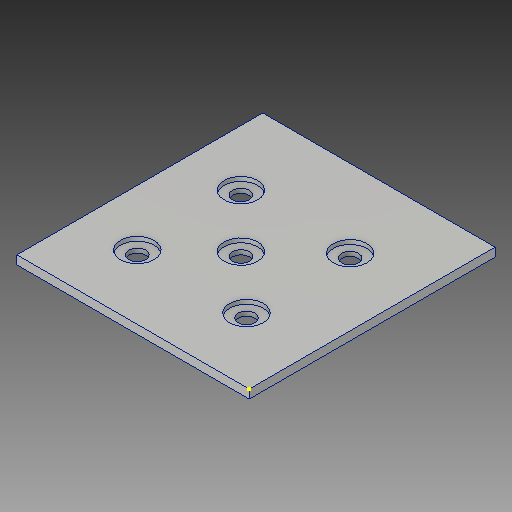
# Autodesk Inventor part: 底板
Saved by Autodesk Inventor 2017 (Build 210142000, 142)
## iProperties
Part Number: 底板
Material: 鋁合金 6061
Document SubType Name: Modeling
Designer: user
Density: 2.7 g/cm^3
Appearance: 鋁 - 平面
Author: user
Autodesk Inventor part; units mm, degrees
ref_plane "YZ Plane" through (0, 0, 0) normal (1, 0, 0) x (0, 1, 0)
ref_plane "XZ Plane" through (0, 0, 0) normal (0, 1, 0) x (-1, 0, 0)
ref_plane "XY Plane" through (0, 0, 0) normal (0, 0, 1) x (1, 0, 0)
sketch "草圖1" plane through (0, 0, 0) normal (0, 1, 0) x (-1, 0, 0)
  line L0 (0, 0) -> (83, 0)
  line L1 (83, 0) -> (83, -87.8)
  line L2 (83, -87.8) -> (0, -87.8)
  line L3 (0, -87.8) -> (0, 0)
  dimension "d0" = 87.8
  dimension "d1" = 83
  constraints: 8 end point, 2 parallel, 1 horizontal, 1 perpendicular
  measures "d0" distance of L0.end L1.end
  measures "d1" distance of L1.end L2.end
extrude "擠出1" add sketch "草圖1" along normal blind 3.1
sketch "草圖2" plane through (0, 3.1, 0) normal (0, 1, 0) x (1, 0, 0)
  line L0 (-24, -18.3432) -> (-24, 108.3328)
  line L1 (-63, -18.3432) -> (-63, 117.1807)
  line L2 (-93.8741, 60) -> (24.8173, 60)
  line L3 (19.8538, 23) -> (-101.6429, 23)
  line L4 (-44, -5.6109) -> (-44, 94.0899)
  line L5 (-89.7738, 41) -> (11.6533, 41)
  line L6 (-83, 0) -> (0, 0) projected
  line L7 (0, 0) -> (0, 87.8) projected
  circle A0 centre (-63, 23) radius 6
  circle A1 centre (-24, 23) radius 6
  circle A2 centre (-24, 60) radius 6
  circle A3 centre (-63, 60) radius 6
  circle A4 centre (-44, 41) radius 6
  dimension "d4" = 23
  dimension "d5" = 37
  dimension "d6" = 24
  dimension "d7" = 44
  dimension "d8" = 39
  dimension "d9" = 41
  dimension "d10" = 12
  dimension "d11" = 12
  dimension "d12" = 12
  dimension "d13" = 12
  dimension "d14" = 12
  constraints: 12 end point, 10 point on line, 5 centre point, 3 horizontal, 3 vertical
  measures "d4" distance between parallel lines of L3 L6
  measures "d5" distance between parallel lines of L2 L3
  measures "d6" distance between parallel lines of L7 L0
  measures "d7" distance between parallel lines of L7 L4
  measures "d8" distance between parallel lines of L0 L1
  measures "d9" distance between parallel lines of L6 L5
  measures "d10" diameter of A0
  measures "d11" diameter of A3
  measures "d12" diameter of A2
  measures "d13" diameter of A1
  measures "d14" diameter of A4
hole "孔1" at (-24, 3.1, -23) at (-63, 3.1, -23) at (-63, 3.1, -60) at (-24, 3.1, -60) direction (0, -1, 0) diameter 6 end through all
sketch "草圖4" plane through (0, 3.1, 0) normal (0, 1, 0) x (1, 0, 0)
  point P0 (0, 0)
sketch "草圖5" plane through (0, 3.1, 0) normal (0, 1, 0) x (1, 0, 0)
  circle A0 centre (-24, 23) radius 3 projected
  circle A1 centre (-24, 23) radius 6
  point P0 (0, 0)
  dimension "d40" = 12
  constraints: 1 centre point, 1 coincident
  measures "d40" diameter of A1
extrude "擠出2" cut sketch "草圖5" against normal blind 1.5
pattern_linear "矩形陣列2" count 2 spacing 39 along (-1, 0, 0) of "擠出2"
sketch "草圖6" plane through (0, 3.1, 0) normal (0, 1, 0) x (1, 0, 0)
  circle A0 centre (-63, 60) radius 3 projected
  circle A1 centre (-63, 60) radius 6
  circle A2 centre (-24, 60) radius 3 projected
  circle A3 centre (-24, 60) radius 6
  point P0 (0, 0)
  dimension "d46" = 12
  dimension "d47" = 12
  constraints: 2 centre point, 2 coincident
  measures "d46" diameter of A3
  measures "d47" diameter of A1
extrude "擠出3" cut sketch "草圖6" against normal blind 1.5
sketch "草圖7" plane through (0, 3.1, 0) normal (0, 1, 0) x (1, 0, 0)
  circle A0 centre (-44, 41) radius 3
  line L0 (-83, 0) -> (0, 0) projected
  line L1 (0, 0) -> (0, 87.8) projected
  dimension "d50" = 6
  dimension "d51" = 41
  dimension "d52" = 44
  constraints: 1 centre point
  measures "d50" diameter of A0
  measures "d51" distance from line of A0.centre L0
  measures "d52" distance from line of A0.centre L1
extrude "擠出4" cut sketch "草圖7" against normal blind 5
sketch "草圖8" plane through (0, 3.1, 0) normal (0, 1, 0) x (1, 0, 0)
  circle A0 centre (-44, 41) radius 3 projected
  circle A1 centre (-44, 41) radius 6
  point P0 (0, 0)
  dimension "d55" = 12
  constraints: 1 centre point, 1 coincident
  measures "d55" diameter of A1
extrude "擠出5" cut sketch "草圖8" against normal blind 1.5
